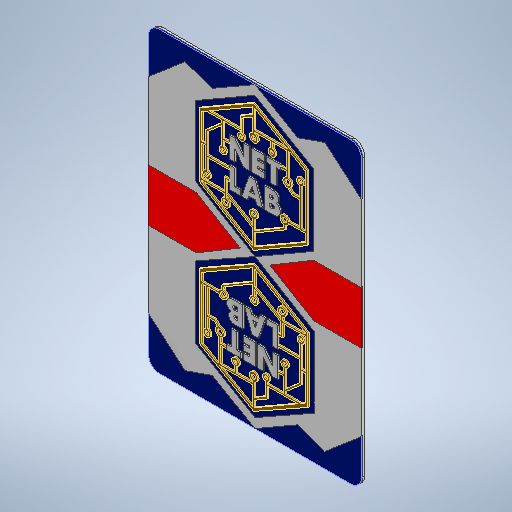
# Autodesk Inventor part: 0ofwifi
Saved by Autodesk Inventor 2025 (Build 290162010, 162A)
## iProperties
Created: 2024-07-12
Part Number: 0ofwifi
Material: Generic
Document SubType Name: Modeling
Designer: joshu
Density: 1 g/cm^3
Appearance: Default
Author: joshu
Autodesk Inventor part; units mm, degrees
(part 1 of 2)
ref_plane "YZ Plane" through (0, 0, 0) normal (1, 0, 0) x (0, 1, 0)
ref_plane "XZ Plane" through (0, 0, 0) normal (0, 1, 0) x (-1, 0, 0)
ref_plane "XY Plane" through (0, 0, 0) normal (0, 0, 1) x (1, 0, 0)
sketch "Sketch1" plane through (0, 0, 0) normal (0, 0, 1) x (1, 0, 0)
  line L0 (0, 0) -> (63.5, 0)
  line L1 (63.5, 0) -> (63.5, 88.9)
  line L2 (63.5, 88.9) -> (0, 88.9)
  line L3 (0, 88.9) -> (0, 0)
  line L4 (31.75, 44.45) -> (49.3079, 54.587)
  line L5 (49.3079, 54.587) -> (49.3079, 75.7826)
  line L6 (49.3079, 75.7826) -> (31.6801, 86.0828)
  line L7 (31.6801, 86.0828) -> (13.967, 75.8563)
  line L8 (13.967, 75.8563) -> (13.967, 55.04)
  line L9 (13.967, 55.04) -> (31.75, 44.45)
  line L10 (15.5263, 74.956) -> (31.6754, 84.2796)
  line L11 (31.6754, 84.2796) -> (47.7487, 74.8877)
  line L12 (47.7487, 74.8877) -> (47.7487, 55.4872)
  line L13 (47.7487, 55.4872) -> (31.7622, 46.2575)
  line L14 (31.7622, 46.2575) -> (15.5263, 55.9263)
  line L15 (15.5263, 55.9263) -> (15.5263, 74.956)
  line L16 (47.1273, 56.0392) -> (31.9379, 47.2671)
  line L17 (31.3664, 47.317) -> (16.2977, 56.192)
  line L18 (41.8086, 77.4972) -> (32.0418, 77.4972)
  line L19 (42.0908, 76.9257) -> (42.0908, 70.0939)
  line L20 (41.5193, 72.1376) -> (39.6994, 72.1376)
  line L21 (39.6994, 72.1376) -> (39.6994, 71.5661)
  line L22 (39.6994, 71.5661) -> (41.5193, 71.5661)
  arc A0 (31.465, 76.5861) -> (32.0365, 76.5861) centre (31.7507, 75.3324) ccw
  arc A1 (36.8763, 75.3571) -> (37.4478, 75.3571) centre (37.162, 74.2504) ccw
  circle A2 centre (37.162, 74.2504) radius 0.4762
  circle A3 centre (31.7507, 75.3324) radius 0.6191
  line L23 (45.9318, 69.8545) -> (45.9318, 58.9507)
  line L24 (45.3603, 66.7769) -> (43.3841, 66.7769)
  line L25 (43.1915, 66.2054) -> (45.3603, 66.2054)
  circle A4 centre (41.805, 68.7917) radius 0.762
  line L26 (43.1915, 66.2054) -> (41.9826, 67.4703)
  line L27 (43.3841, 66.7769) -> (42.5287, 67.6719)
  arc A5 (45.9318, 69.8545) -> (45.3603, 69.8545) centre (45.646, 70.9598) ccw
  circle A6 centre (45.646, 70.9598) radius 0.5715
  line L28 (40.6132, 56.5528) -> (40.6132, 57.4113)
  circle A7 centre (40.899, 58.665) radius 0.7144
  line L29 (32.0418, 83.1688) -> (32.0418, 77.4972)
  line L30 (32.0365, 76.9257) -> (32.0365, 76.5861)
  line L31 (32.0365, 76.9257) -> (36.8763, 76.9257)
  line L32 (36.8763, 75.3571) -> (36.8763, 76.9257)
  line L33 (37.4478, 76.9257) -> (37.4478, 75.3571)
  line L34 (37.4478, 76.9257) -> (41.5193, 76.9257)
  line L35 (42.0908, 76.9257) -> (42.7928, 76.9257)
  line L36 (32.0365, 83.1719) -> (41.8086, 77.4972)
  line L37 (42.7928, 76.9257) -> (47.1273, 74.4086)
  line L38 (41.5193, 70.0939) -> (41.5193, 71.5661)
  line L39 (41.5193, 72.1376) -> (41.5193, 76.9257)
  arc A8 (41.5193, 70.0939) -> (41.9826, 67.4703) centre (41.805, 68.7917) ccw
  arc A9 (42.5287, 67.6719) -> (42.0908, 70.0939) centre (41.805, 68.7917) ccw
  line L40 (45.3603, 58.9507) -> (45.3603, 66.2054)
  line L41 (45.3603, 66.7769) -> (45.3603, 69.8545)
  line L42 (47.1273, 58.9507) -> (45.9318, 58.9507)
  line L43 (45.3603, 58.9507) -> (42.1527, 58.9507)
  line L44 (42.1475, 58.3804) -> (47.1273, 58.3804)
  line L45 (41.1819, 57.4161) -> (41.1819, 56.2658)
  arc A10 (42.1527, 58.9507) -> (40.6132, 57.4113) centre (40.899, 58.665) ccw
  arc A11 (41.1819, 57.4161) -> (42.1475, 58.3804) centre (40.899, 58.665) ccw
  line L46 (47.1273, 74.4086) -> (47.1273, 58.9507)
  line L47 (47.1273, 58.3804) -> (47.1273, 56.0392)
  line L48 (27.6974, 78.6822) -> (27.6974, 79.0777)
  line L49 (28.2689, 78.6822) -> (31.465, 80.528)
  line L50 (27.6974, 79.0777) -> (31.465, 81.2535)
  line L51 (31.465, 76.5861) -> (31.465, 80.528)
  line L52 (31.465, 81.2535) -> (31.465, 83.1596)
  line L53 (31.9379, 51.4601) -> (40.6132, 56.5528)
  line L54 (31.9379, 50.8392) -> (41.1819, 56.2658)
  line L55 (16.2977, 57.1448) -> (22.9994, 57.1448)
  line L56 (22.9994, 56.5733) -> (16.2977, 56.5733)
  line L57 (16.2977, 56.5733) -> (16.2977, 57.1448)
  line L58 (22.9994, 60.9472) -> (23.5709, 60.9472)
  line L59 (22.9994, 60.9472) -> (24.4329, 60.9472)
  line L60 (24.4329, 60.9472) -> (24.4329, 60.3757)
  line L61 (24.4329, 60.3757) -> (23.5709, 60.3757)
  line L62 (22.9994, 60.3757) -> (22.9994, 60.9472)
  line L63 (23.5709, 56.4373) -> (31.3664, 51.9861)
  line L64 (31.3664, 52.5972) -> (23.5709, 57.0484)
  arc A12 (31.9379, 54.3552) -> (31.3664, 54.3552) centre (31.6521, 55.5111) ccw
  circle A13 centre (31.6521, 55.5111) radius 0.6191
  arc A14 (22.9994, 55.5805) -> (23.5709, 55.5805) centre (23.2852, 54.3309) ccw
  circle A15 centre (23.2852, 54.3309) radius 0.7144
  line L65 (23.5709, 60.3757) -> (23.5709, 57.0484)
  line L66 (23.5709, 56.4373) -> (23.5709, 55.5805)
  line L67 (22.9994, 55.5805) -> (22.9994, 56.5733)
  line L68 (22.9994, 57.1448) -> (22.9994, 60.9472)
  line L69 (31.3664, 54.3552) -> (31.3664, 52.5972)
  line L70 (31.3664, 51.9861) -> (31.3664, 47.317)
  line L71 (31.9379, 47.2671) -> (31.9379, 50.8392)
  line L72 (31.9379, 51.4601) -> (31.9379, 54.3552)
  arc A16 (27.6974, 74.6924) -> (28.2689, 74.6924) centre (27.9831, 73.6844) ccw
  circle A17 centre (27.9831, 73.6844) radius 0.4763
  line L73 (18.5492, 75.7007) -> (27.6974, 75.7007)
  line L74 (22.769, 70.6818) -> (24.4329, 70.6818)
  line L75 (24.4329, 70.6818) -> (24.4329, 70.1103)
  line L76 (24.4329, 70.1103) -> (22.769, 70.1103)
  line L77 (22.769, 70.1103) -> (22.769, 70.2009)
  line L78 (16.2977, 66.7769) -> (17.4065, 66.7769)
  line L79 (17.978, 66.7769) -> (17.978, 66.2054)
  line L80 (17.4065, 66.2054) -> (16.2977, 66.2054)
  line L81 (17.978, 63.9706) -> (24.4329, 63.9706)
  line L82 (24.4329, 63.9706) -> (24.4329, 63.3991)
  line L83 (24.4329, 63.3991) -> (17.978, 63.3991)
  line L84 (17.4065, 66.7769) -> (17.4065, 70.2549)
  line L85 (17.978, 70.0307) -> (17.978, 66.7769)
  line L86 (17.4065, 70.2549) -> (22.1975, 74.4365)
  line L87 (17.978, 70.0307) -> (22.1975, 73.7135)
  arc A18 (22.1975, 68.5281) -> (22.769, 68.5281) centre (22.4833, 67.4703) ccw
  circle A19 centre (22.4833, 67.4703) radius 0.5239
  line L88 (16.2977, 74.4004) -> (17.5596, 75.1292)
  line L89 (18.5492, 75.7007) -> (31.465, 83.1596)
  line L90 (27.6974, 75.1292) -> (22.769, 75.1292)
  line L91 (22.1975, 75.1292) -> (17.5596, 75.1292)
  line L92 (22.1975, 74.4365) -> (22.1975, 75.1292)
  line L93 (28.2689, 74.6924) -> (28.2689, 78.6822)
  line L94 (22.769, 75.1292) -> (22.769, 70.6818)
  line L95 (22.769, 70.1103) -> (22.769, 68.5281)
  line L96 (22.1975, 67.8875) -> (22.1975, 67.9094)
  line L97 (22.1975, 68.5281) -> (22.1975, 73.7135)
  line L98 (16.2977, 56.192) -> (16.2977, 66.2054)
  line L99 (16.2977, 66.7769) -> (16.2977, 74.4004)
  line L100 (17.978, 63.9706) -> (17.978, 66.2054)
  line L101 (27.6974, 78.6822) -> (27.6974, 75.7007)
  line L102 (27.6974, 75.1292) -> (27.6974, 74.6924)
  line L103 (24.4329, 66.1976) -> (26.1474, 66.1976)
  line L104 (26.1474, 66.1976) -> (26.1474, 69.7075)
  line L105 (26.1474, 72.4542) -> (24.4329, 72.4542)
  line L106 (24.4329, 72.4542) -> (24.4329, 66.1976)
  line L107 (28.7777, 72.4542) -> (30.4922, 72.4542)
  line L108 (30.4922, 72.4542) -> (30.4922, 66.1976)
  line L109 (30.4922, 66.1976) -> (28.7777, 66.1976)
  line L110 (28.7777, 68.9443) -> (28.7777, 72.4542)
  line L111 (28.7777, 66.1976) -> (26.1474, 69.7075)
  line L112 (26.1474, 72.4542) -> (28.7777, 68.9443)
  line L113 (31.2537, 72.4542) -> (32.9682, 72.4542)
  line L114 (32.9682, 66.1976) -> (31.2537, 66.1976)
  line L115 (31.2537, 66.1976) -> (31.2537, 72.4542)
  line L116 (31.2537, 72.4542) -> (34.8385, 72.4542)
  line L117 (34.8385, 72.4542) -> (34.8385, 70.7397)
  line L118 (34.8385, 70.7397) -> (32.9682, 70.7397)
  line L119 (31.2537, 70.7397) -> (31.2537, 72.4542)
  line L120 (32.9682, 70.0633) -> (34.8385, 70.0633)
  line L121 (34.8385, 70.0633) -> (34.8385, 68.5393)
  line L122 (34.8385, 68.5393) -> (32.9682, 68.5393)
  line L123 (31.2537, 68.5393) -> (31.2537, 70.0633)
  line L124 (31.2537, 66.1976) -> (34.8385, 66.1976)
  line L125 (34.8385, 66.1976) -> (34.8385, 67.9121)
  line L126 (34.8385, 67.9121) -> (32.9682, 67.9121)
  line L127 (31.2537, 67.9121) -> (31.2537, 66.1976)
  line L128 (32.9682, 70.7397) -> (32.9682, 70.0633)
  line L129 (32.9682, 68.5393) -> (32.9682, 67.9121)
  line L130 (39.6994, 72.4422) -> (35.4849, 72.4422)
  line L131 (35.4849, 72.4422) -> (35.4849, 70.9182)
  line L132 (39.6994, 70.9182) -> (39.6994, 72.4422)
  line L133 (38.4466, 70.9182) -> (38.4466, 66.1976)
  line L134 (38.4466, 66.1976) -> (36.7321, 66.1976)
  line L135 (36.7321, 66.1976) -> (36.7321, 70.9182)
  line L136 (36.7321, 70.9182) -> (36.8763, 70.9182)
  line L137 (35.4849, 70.9182) -> (36.7321, 70.9182)
  line L138 (38.4466, 70.9182) -> (39.6994, 70.9182)
  line L139 (24.4329, 64.6461) -> (26.1474, 64.6461)
  line L140 (26.1474, 64.6461) -> (26.1474, 59.9044)
  line L141 (26.1474, 58.3804) -> (24.4329, 58.3804)
  line L142 (24.4329, 58.3804) -> (24.4329, 64.6461)
  line L143 (24.4329, 58.3804) -> (27.8234, 58.3804)
  line L144 (27.8234, 58.3804) -> (27.8234, 59.9044)
  line L145 (27.8234, 59.9044) -> (26.1474, 59.9044)
  line L146 (24.4329, 59.9044) -> (24.4329, 58.3804)
  line L147 (28.1466, 58.3804) -> (29.8611, 58.3804)
  line L148 (29.8611, 58.3804) -> (30.3254, 59.5144)
  line L149 (30.3254, 59.5144) -> (32.2304, 59.5144)
  line L150 (30.3254, 64.6461) -> (32.2304, 64.6461)
  line L151 (28.1466, 58.3804) -> (30.3254, 64.6461)
  line L152 (32.728, 58.3804) -> (34.4425, 58.3804)
  line L153 (32.728, 58.3804) -> (32.2304, 59.5144)
  line L154 (34.4425, 58.3804) -> (32.2304, 64.6461)
  line L155 (30.6203, 60.8236) -> (31.9379, 60.8236)
  line L156 (31.9379, 60.8236) -> (31.2779, 62.4085)
  line L157 (31.2779, 62.4085) -> (30.6203, 60.8236)
  line L158 (34.9216, 58.3804) -> (34.9216, 64.6461)
  line L159 (34.9216, 64.6461) -> (37.8691, 64.6461)
  line L160 (34.9216, 58.3804) -> (37.8691, 58.3804)
  line L161 (36.5599, 59.8143) -> (36.5599, 60.939)
  line L162 (36.5599, 62.1736) -> (36.5599, 63.1944)
  line L163 (36.5599, 63.1944) -> (37.2133, 63.1944)
  line L164 (36.5599, 62.1736) -> (37.2133, 62.1736)
  arc A20 (37.2133, 62.1736) -> (37.2133, 63.1944) centre (37.055, 62.684) ccw
  line L165 (36.5599, 60.939) -> (37.4519, 60.939)
  line L166 (36.5599, 59.8143) -> (37.4396, 59.8143)
  arc A21 (37.4396, 59.8143) -> (37.4519, 60.939) centre (37.3959, 60.3772) ccw
  arc A22 (38.5631, 61.7817) -> (37.8691, 64.6461) centre (37.5266, 63.0469) ccw
  arc A23 (37.8691, 58.3804) -> (38.5631, 61.7817) centre (37.9604, 60.1332) ccw
  arc A24 (17.4065, 59.8724) -> (17.978, 59.8724) centre (17.6923, 58.815) ccw
  circle A25 centre (17.6923, 58.815) radius 0.5239
  line L167 (17.4065, 66.2054) -> (17.4065, 59.8724)
  line L168 (17.978, 59.8724) -> (17.978, 63.3991)
  line L169 (32.0418, 83.1688) -> (41.8086, 77.4972)
  line L170 (32.0418, 77.4972) -> (41.8086, 77.4972)
  line L171 (32.0418, 77.4972) -> (32.0418, 83.1688)
  line L172 (0, 44.45) -> (63.5, 44.45) construction
  line L173 (31.75, 88.9) -> (31.75, 0) construction
  line L174 (0, 52.2573) -> (14.2102, 52.2573)
  line L175 (14.2102, 52.2573) -> (27.3204, 44.45)
  line L176 (0, 36.6427) -> (14.2102, 36.6427)
  line L177 (14.2102, 36.6427) -> (27.3204, 44.45)
  line L178 (63.5, 52.2573) -> (49.2898, 52.2573)
  line L179 (49.2898, 52.2573) -> (36.1796, 44.45)
  line L180 (49.2898, 36.6427) -> (36.1796, 44.45)
  line L181 (63.5, 36.6427) -> (49.2898, 36.6427)
  line L182 (0, 75.0796) -> (10.8905, 84.3747)
  line L183 (10.8905, 84.3747) -> (18.9583, 81.5148)
  line L184 (18.9583, 81.5148) -> (31.75, 88.9)
  line L185 (63.5, 75.0796) -> (52.6095, 84.3747)
  line L186 (52.6095, 84.3747) -> (44.5417, 81.5148)
  line L187 (44.5417, 81.5148) -> (31.75, 88.9)
  line L188 (46.0393, 22.6946) -> (47.1481, 22.6946)
  line L189 (45.4678, 22.1231) -> (45.4678, 22.6946)
  line L190 (45.4678, 24.9294) -> (45.4678, 22.6946)
  line L191 (47.1481, 22.1231) -> (46.0393, 22.1231)
  line L192 (47.1481, 32.3267) -> (47.1481, 31.7552)
  line L193 (47.1481, 32.708) -> (47.1481, 22.6946)
  line L194 (47.1481, 31.7552) -> (40.4464, 31.7552)
  line L195 (40.4464, 32.3267) -> (47.1481, 32.3267)
  line L196 (45.4678, 29.0276) -> (45.4678, 25.5009)
  line L197 (46.0393, 22.6946) -> (46.0393, 29.0276)
  circle A26 centre (45.7535, 30.085) radius 0.5239
  arc A27 (46.0393, 29.0276) -> (45.4678, 29.0276) centre (45.7535, 30.085) ccw
  line L198 (20.6531, 11.9743) -> (16.3185, 14.4914)
  line L199 (21.355, 11.9743) -> (20.6531, 11.9743)
  line L200 (21.9265, 16.7624) -> (21.9265, 11.9743)
  line L201 (21.355, 11.9743) -> (21.355, 18.8061)
  line L202 (21.9265, 16.7624) -> (23.7464, 16.7624)
  line L203 (23.7464, 17.3339) -> (21.9265, 17.3339)
  line L204 (25.998, 11.9743) -> (21.9265, 11.9743)
  line L205 (26.5695, 13.5429) -> (26.5695, 11.9743)
  circle A28 centre (21.6408, 20.1083) radius 0.762
  circle A29 centre (26.2838, 14.6496) radius 0.4762
  arc A30 (26.5695, 13.5429) -> (25.998, 13.5429) centre (26.2838, 14.6496) ccw
  line L206 (31.4093, 11.9743) -> (26.5695, 11.9743)
  arc A31 (31.9808, 12.3139) -> (31.4093, 12.3139) centre (31.6951, 13.5676) ccw
  line L207 (25.998, 11.9743) -> (25.998, 13.5429)
  line L208 (45.4678, 24.9294) -> (39.013, 24.9294)
  line L209 (39.013, 25.5009) -> (45.4678, 25.5009)
  line L210 (39.013, 24.9294) -> (39.013, 25.5009)
  circle A32 centre (40.1606, 34.5691) radius 0.7144
  arc A33 (40.4464, 33.3195) -> (39.8749, 33.3195) centre (40.1606, 34.5691) ccw
  line L211 (39.8749, 32.4627) -> (39.8749, 33.3195)
  line L212 (40.4464, 33.3195) -> (40.4464, 32.3267)
  line L213 (39.013, 27.9528) -> (39.013, 28.5243)
  line L214 (39.8749, 28.5243) -> (39.8749, 31.8516)
  line L215 (39.013, 28.5243) -> (39.8749, 28.5243)
  line L216 (40.4464, 31.7552) -> (40.4464, 27.9528)
  line L217 (40.4464, 28.5243) -> (40.4464, 27.9528)
  line L218 (40.4464, 27.9528) -> (39.8749, 27.9528)
  line L219 (40.4464, 27.9528) -> (39.013, 27.9528)
  line L220 (33.5847, 30.5196) -> (33.1204, 29.3856)
  line L221 (35.6224, 28.9956) -> (37.2985, 28.9956)
  line L222 (35.2992, 30.5196) -> (33.5847, 30.5196)
  line L223 (39.013, 28.9956) -> (39.013, 30.5196)
  line L224 (35.2992, 30.5196) -> (33.1204, 24.2539)
  line L225 (46.0393, 18.6451) -> (41.2483, 14.4635)
  line L226 (45.4678, 18.8693) -> (41.2483, 15.1865)
  line L227 (40.6768, 18.7897) -> (40.6768, 20.3719)
  line L228 (41.2483, 21.0125) -> (41.2483, 20.9906)
  line L229 (41.2483, 20.3719) -> (41.2483, 15.1865)
  line L230 (40.6768, 13.7708) -> (40.6768, 18.2182)
  line L231 (41.2483, 14.4635) -> (41.2483, 13.7708)
  line L232 (41.2483, 13.7708) -> (45.8862, 13.7708)
  line L233 (47.1481, 22.1231) -> (47.1481, 14.4996)
  line L234 (47.1481, 14.4996) -> (45.8862, 13.7708)
  circle A34 centre (40.9626, 21.4297) radius 0.5239
  line L235 (32.8255, 28.0764) -> (31.5079, 28.0764)
  line L236 (32.1679, 26.4915) -> (32.8255, 28.0764)
  line L237 (31.5079, 28.0764) -> (32.1679, 26.4915)
  line L238 (33.1204, 29.3856) -> (31.2154, 29.3856)
  line L239 (35.6224, 30.5196) -> (35.6224, 28.9956)
  line L240 (37.2985, 24.2539) -> (37.2985, 28.9956)
  line L241 (37.2985, 30.5196) -> (39.013, 30.5196)
  line L242 (39.013, 30.5196) -> (39.013, 24.2539)
  line L243 (39.013, 30.5196) -> (35.6224, 30.5196)
  line L244 (39.013, 24.2539) -> (37.2985, 24.2539)
  line L245 (33.1204, 24.2539) -> (31.2154, 24.2539)
  line L246 (30.7178, 30.5196) -> (31.2154, 29.3856)
  line L247 (37.2985, 16.4458) -> (39.013, 16.4458)
  line L248 (40.6768, 18.2182) -> (39.013, 18.2182)
  line L249 (39.013, 18.7897) -> (40.6768, 18.7897)
  line L250 (40.6768, 18.7897) -> (40.6768, 18.6991)
  line L251 (39.013, 18.2182) -> (39.013, 18.7897)
  line L252 (46.0393, 22.1231) -> (46.0393, 18.6451)
  line L253 (45.4678, 18.8693) -> (45.4678, 22.1231)
  arc A35 (41.2483, 20.3719) -> (40.6768, 20.3719) centre (40.9626, 21.4297) ccw
  line L254 (39.013, 16.4458) -> (39.013, 22.7024)
  line L255 (39.013, 22.7024) -> (37.2985, 22.7024)
  line L256 (32.9536, 22.7024) -> (34.6681, 22.7024)
  line L257 (30.4777, 22.7024) -> (32.1922, 22.7024)
  line L258 (30.4777, 18.8367) -> (28.6073, 18.8367)
  line L259 (32.1922, 22.7024) -> (28.6073, 22.7024)
  line L260 (28.6073, 22.7024) -> (28.6073, 20.9879)
  line L261 (28.6073, 20.9879) -> (30.4777, 20.9879)
  line L262 (32.1922, 20.9879) -> (32.1922, 22.7024)
  line L263 (30.4777, 20.3607) -> (30.4777, 20.9879)
  line L264 (28.6073, 20.3607) -> (30.4777, 20.3607)
  line L265 (28.6073, 18.8367) -> (28.6073, 20.3607)
  line L266 (32.1922, 20.3607) -> (32.1922, 18.8367)
  line L267 (30.4777, 18.1603) -> (30.4777, 18.8367)
  line L268 (26.8859, 25.7056) -> (26.2325, 25.7056)
  line L269 (26.8859, 29.0857) -> (26.0062, 29.0857)
  line L270 (26.8859, 27.961) -> (25.9939, 27.961)
  line L271 (28.5242, 30.5196) -> (25.5767, 30.5196)
  line L272 (32.0794, 36.9139) -> (32.0794, 41.583)
  line L273 (31.5079, 41.6329) -> (31.5079, 38.0608)
  line L274 (26.8859, 26.7264) -> (26.8859, 25.7056)
  line L275 (28.5242, 24.2539) -> (25.5767, 24.2539)
  line L276 (29.0033, 30.5196) -> (31.2154, 24.2539)
  line L277 (30.7178, 30.5196) -> (29.0033, 30.5196)
  line L278 (26.8859, 26.7264) -> (26.2325, 26.7264)
  line L279 (28.5242, 30.5196) -> (28.5242, 24.2539)
  arc A36 (26.2325, 26.7264) -> (26.2325, 25.7056) centre (26.3908, 26.216) ccw
  line L280 (26.8859, 29.0857) -> (26.8859, 27.961)
  arc A37 (26.0062, 29.0857) -> (25.9939, 27.961) centre (26.0499, 28.5228) ccw
  arc A38 (24.8827, 27.1183) -> (25.5767, 24.2539) centre (25.9192, 25.8531) ccw
  arc A39 (25.5767, 30.5196) -> (24.8827, 27.1183) centre (25.4854, 28.7668) ccw
  line L281 (23.7464, 16.7624) -> (23.7464, 17.3339)
  line L282 (24.9992, 22.7024) -> (26.7137, 22.7024)
  line L283 (27.961, 17.9818) -> (26.7137, 17.9818)
  line L284 (26.7137, 22.7024) -> (26.7137, 17.9818)
  line L285 (26.7137, 17.9818) -> (26.5695, 17.9818)
  line L286 (24.9992, 17.9818) -> (24.9992, 22.7024)
  line L287 (24.9992, 17.9818) -> (23.7464, 17.9818)
  line L288 (27.961, 16.4578) -> (27.961, 17.9818)
  line L289 (23.7464, 16.4578) -> (27.961, 16.4578)
  line L290 (23.7464, 17.9818) -> (23.7464, 16.4578)
  line L291 (31.75, 44.45) -> (14.1379, 34.5158)
  line L292 (15.6972, 33.6051) -> (31.7276, 42.6471)
  line L293 (16.3185, 32.8608) -> (31.5079, 41.6329)
  line L294 (31.5079, 37.4399) -> (22.8326, 32.3472)
  line L295 (31.5079, 38.0608) -> (22.2639, 32.6342)
  line L296 (31.5079, 37.4399) -> (31.5079, 34.5448)
  line L297 (35.7484, 10.2178) -> (35.7484, 9.8223)
  line L298 (35.1769, 10.2178) -> (31.9808, 8.372)
  line L299 (35.7484, 9.8223) -> (31.9808, 7.6465)
  line L300 (31.9808, 12.3139) -> (31.9808, 8.372)
  line L301 (31.9808, 7.6465) -> (31.9808, 5.7404)
  circle A40 centre (35.4627, 15.2156) radius 0.4763
  arc A41 (35.7484, 14.2076) -> (35.1769, 14.2076) centre (35.4627, 15.2156) ccw
  line L302 (35.7484, 13.7708) -> (35.7484, 14.2076)
  line L303 (35.7484, 13.7708) -> (40.6768, 13.7708)
  line L304 (44.8966, 13.1993) -> (35.7484, 13.1993)
  line L305 (35.1769, 14.2076) -> (35.1769, 10.2178)
  line L306 (35.7484, 10.2178) -> (35.7484, 13.1993)
  line L307 (44.8966, 13.1993) -> (31.9808, 5.7404)
  line L308 (31.4093, 11.9743) -> (31.4093, 12.3139)
  line L309 (47.9195, 13.7706) -> (31.7623, 4.657)
  circle A42 centre (31.6951, 13.5676) radius 0.6191
  line L310 (31.7499, 2.8598) -> (49.4788, 12.8599)
  line L311 (47.9195, 32.9751) -> (47.9195, 13.7706)
  line L312 (49.4788, 12.8599) -> (49.4788, 33.86)
  circle A43 centre (31.7937, 33.3889) radius 0.6191
  line L313 (32.0794, 41.583) -> (47.1481, 32.708)
  line L314 (49.4788, 33.86) -> (31.75, 44.45)
  line L315 (31.7276, 42.6471) -> (47.9195, 32.9751)
  line L316 (32.0794, 36.3028) -> (39.8749, 31.8516)
  line L317 (39.8749, 32.4627) -> (32.0794, 36.9139)
  line L318 (32.0794, 34.5448) -> (32.0794, 36.3028)
  arc A44 (31.5079, 34.5448) -> (32.0794, 34.5448) centre (31.7937, 33.3889) ccw
  circle A45 centre (17.7998, 17.9402) radius 0.5715
  line L319 (18.0855, 22.1231) -> (20.0617, 22.1231)
  line L320 (20.2543, 22.6946) -> (18.0855, 22.6946)
  line L321 (22.8326, 32.3472) -> (22.8326, 31.4887)
  circle A46 centre (22.5468, 30.235) radius 0.7144
  line L322 (21.2984, 30.5196) -> (16.3185, 30.5196)
  line L323 (22.2639, 31.4839) -> (22.2639, 32.6342)
  arc A47 (21.2931, 29.9493) -> (22.8326, 31.4887) centre (22.5468, 30.235) ccw
  arc A48 (22.2639, 31.4839) -> (21.2984, 30.5196) centre (22.5468, 30.235) ccw
  line L324 (16.3185, 30.5196) -> (16.3185, 32.8608)
  line L325 (14.1379, 34.5158) -> (14.1379, 13.1174)
  line L326 (15.6972, 14.0137) -> (15.6972, 33.6051)
  line L327 (17.514, 19.0455) -> (17.514, 29.9493)
  line L328 (20.2543, 22.6946) -> (21.4633, 21.4297)
  line L329 (20.0617, 22.1231) -> (20.9171, 21.2281)
  arc A49 (17.514, 19.0455) -> (18.0855, 19.0455) centre (17.7998, 17.9402) ccw
  line L330 (21.9265, 18.8061) -> (21.9265, 17.3339)
  arc A50 (20.9171, 21.2281) -> (21.355, 18.8061) centre (21.6408, 20.1083) ccw
  line L331 (18.0855, 22.1231) -> (18.0855, 19.0455)
  line L332 (16.3185, 14.4914) -> (16.3185, 29.9493)
  line L333 (16.3185, 29.9493) -> (17.514, 29.9493)
  line L334 (18.0855, 29.9493) -> (18.0855, 22.6946)
  line L335 (18.0855, 29.9493) -> (21.2931, 29.9493)
  arc A51 (21.9265, 18.8061) -> (21.4633, 21.4297) centre (21.6408, 20.1083) ccw
  line L336 (14.1379, 13.1174) -> (31.7499, 2.8598)
  line L337 (31.7623, 4.657) -> (15.6972, 14.0137)
  line L338 (21.6372, 11.4028) -> (31.404, 11.4028)
  line L339 (31.404, 11.4028) -> (31.404, 5.7312)
  line L340 (31.404, 5.7312) -> (21.6372, 11.4028)
  line L341 (37.2985, 22.7024) -> (37.2985, 19.1925)
  line L342 (34.6681, 16.4458) -> (32.9536, 16.4458)
  line L343 (32.9536, 16.4458) -> (32.9536, 22.7024)
  line L344 (34.6681, 22.7024) -> (37.2985, 19.1925)
  line L345 (28.6073, 18.1603) -> (30.4777, 18.1603)
  line L346 (32.1922, 16.4458) -> (28.6073, 16.4458)
  line L347 (28.6073, 16.4458) -> (28.6073, 18.1603)
  line L348 (32.1922, 22.7024) -> (32.1922, 16.4458)
  line L349 (32.1922, 16.4458) -> (30.4777, 16.4458)
  line L350 (34.6681, 19.9557) -> (34.6681, 16.4458)
  line L351 (37.2985, 16.4458) -> (34.6681, 19.9557)
  line L352 (32.1922, 18.1603) -> (32.1922, 16.4458)
  line L353 (0, 13.8204) -> (10.8905, 4.5253)
  line L354 (10.8905, 4.5253) -> (18.9583, 7.3852)
  line L355 (18.9583, 7.3852) -> (31.75, 0)
  line L356 (63.5, 13.8204) -> (52.6095, 4.5253)
  line L357 (52.6095, 4.5253) -> (44.5417, 7.3852)
  line L358 (44.5417, 7.3852) -> (31.75, 0)
  point P0 (31.9379, 47.317)
  point P1 (31.7229, 65.2666)
  point P2 (31.7229, 23.6334)
  point P3 (31.7229, 23.6334)
  point P4 (31.9379, 5.6837)
  point P5 (63.5, 75.0796)
  dimension "d0" = 63.5
  dimension "d1" = 88.9
  dimension "d43" = 44.45
  dimension "d99" = 120
  constraints: 718 end point, 170 parallel, 64 point on circle, 50 centre point, 42 perpendicular, 36 horizontal, 21 point on line, 20 coincident, 19 symmetric about line, 7 collinear, 5 midpoint, 4 vertical, 17 other
  measures "d0" distance of L2.end L1.end
  measures "d1" distance of L1.end L0.end
  measures "d43" distance between parallel lines of L172 L2
  measures "d99" angle of L357 L356
extrude "Extrusion1" add sketch "Sketch1" along normal blind 0.4 contours L3 L353 L354 L355 L0 | L358 L357 L356 L1 L0 | L3 L2 L184 L183 L182 | L185 L186 L187 L2 L1 | L9 L8 L7 L6 L5 L4 | L314 L312 L310 L336 L325 L291 | L10 L11 L12 L13 L14 L15 | L16 L71 L54 L45 A11 L44 L47 | L17 L98 L56 L67 A14 L66 L63 L70 | L18 L29 L36 | L35 L37 L46 L42 L23 A5 L41 L24 L27 A9 L19 | L20 L132 L130 L131 L137 L135 L134 L133 L138 L22 L38 A8 L26 L25 L40 L43 A10 L28 L53 L72 A12 L69 L64 L65 L61 L142 L141 L143 L144 L145 L140 L139 L81 L100 L79 L85 L87 L97 A18 L95 L76 L106 L103 L104 L111 L109 L108 L107 L110 L112 L105 L74 L94 L90 L102 A16 L93 L49 L51 A0 L30 L31 L32 A1 L33 L34 L39 | L21 L132 L138 L133 L134 L135 L137 L131 L130 | L106 L105 L112 L110 L107 L108 L109 L111 L104 L103 L75 | L60 L142 L82 L139 L140 L145 L144 L143 L141 | L59 L58 L62 L68 L55 L98 L80 L167 A24 L168 L83 L142 | A2 | A3 | A4 | A6 | A7 | L101 L73 L89 L52 L50 L48 | A13 | A15 | A17 | L99 L88 L91 L92 L86 L84 L78 | A19 | L113 L116 L117 L118 L128 L120 L121 L122 L129 L126 L125 L124 L114 L115 | L151 L150 L154 L152 L153 L149 L148 L147 | L157 L156 L155 | L158 L159 A22 A23 L160 | L161 L165 A21 L166 | L162 L163 A20 L164 | A25 | L197 A27 L196 L209 L242 L219 L218 L216 L194 L193 L188 | L210 L242 L244 L240 L221 L239 L243 L241 L223 L213 | L208 L190 L189 L253 L226 L229 A35 L227 L249 L254 L255 L341 L344 L256 L343 L342 L350 L351 L247 L248 L230 L303 L302 A41 L305 L298 L300 A31 L308 L206 L205 A30 L207 L204 L200 L202 L290 L289 L288 L283 L284 L282 L286 L287 L203 L330 A51 L328 L320 L334 L335 A47 L321 L294 L296 A44 L318 L316 L214 L215 L242 L223 L241 L243 L239 L221 L240 L244 | L251 L254 L247 L351 L350 L342 L343 L256 L344 L341 L255 | L290 L287 L286 L282 L284 L283 L288 L289 L281 | L233 L234 L232 L231 L225 L252 L191 | L193 L195 L212 A33 L211 L317 L272 L313 | A26 | L198 L332 L333 L327 A49 L331 L319 L329 A50 L201 L199 | A28 | A29 | A32 | L222 L224 L245 L276 L277 L246 L238 L220 | A34 | L236 L237 L235 | L257 L262 L348 L266 L346 L347 L345 L267 L258 L265 L264 L263 L261 L260 L259 | L268 A36 L278 L274 | L280 L270 A37 L269 | L279 L275 A38 A39 L271 | L273 L295 L323 A48 L322 L324 L293 | L292 L315 L311 L309 L337 L326 | L306 L304 L307 L301 L299 L297 | A40 | A42 | A43 | A45 | A46 | L338 L339 L340
extrude "Extrusion12" add sketch "Sketch1" along normal blind 0.4 separate body contours L3 L174 L175 L177 L176 | L181 L180 L179 L178 L1
extrude "Extrusion13" add sketch "Sketch1" along normal blind 0.4 separate body contours L355 L354 L353 L3 L176 L177 L175 L174 L182 L183 L184 L187 L186 L185 L1 L178 L179 L180 L181 L356 L357 L358
extrude "Extrusion14" add sketch "Sketch1" against normal blind 0.4 contours L21 L132 L138 L133 L134 L135 L137 L131 L130 | L106 L105 L112 L110 L107 L108 L109 L111 L104 L103 L75 | L60 L142 L82 L139 L140 L145 L144 L143 L141 | L113 L116 L117 L118 L128 L120 L121 L122 L129 L126 L125 L124 L114 L115 | L151 L150 L154 L152 L153 L149 L148 L147 | L158 L159 A22 A23 L160 | L210 L242 L244 L240 L221 L239 L243 L241 L223 L213 | L251 L254 L247 L351 L350 L342 L343 L256 L344 L341 L255 | L290 L287 L286 L282 L284 L283 L288 L289 L281 | L222 L224 L245 L276 L277 L246 L238 L220 | L257 L262 L348 L266 L346 L347 L345 L267 L258 L265 L264 L263 L261 L260 L259 | L279 L275 A38 A39 L271 bodies 3
extrude "Extrusion15" add sketch "Sketch1" against normal blind 0.4 separate body contours L10 L11 L12 L13 L14 L15 | L292 L315 L311 L309 L337 L326
pattern_linear "Rectangular Pattern1" count 2 spacing 0.8 along (0, 0, 1) of "Extrusion15" bodies 4
pattern_linear "Rectangular Pattern2" count 2 spacing 0.8 along (0, 0, 1) of "Extrusion14" bodies 3
extrude "Extrusion16" cut sketch "Sketch1" against normal blind 0.4 contours L9 L8 L7 L6 L5 L4 | L314 L312 L310 L336 L325 L291 | L10 L11 L12 L13 L14 L15 | L16 L71 L54 L45 A11 L44 L47 | L17 L98 L56 L67 A14 L66 L63 L70 | L18 L29 L36 | L35 L37 L46 L42 L23 A5 L41 L24 L27 A9 L19 | L20 L132 L130 L131 L137 L135 L134 L133 L138 L22 L38 A8 L26 L25 L40 L43 A10 L28 L53 L72 A12 L69 L64 L65 L61 L142 L141 L143 L144 L145 L140 L139 L81 L100 L79 L85 L87 L97 A18 L95 L76 L106 L103 L104 L111 L109 L108 L107 L110 L112 L105 L74 L94 L90 L102 A16 L93 L49 L51 A0 L30 L31 L32 A1 L33 L34 L39 | L21 L132 L138 L133 L134 L135 L137 L131 L130 | L106 L105 L112 L110 L107 L108 L109 L111 L104 L103 L75 | L60 L142 L82 L139 L140 L145 L144 L143 L141 | L59 L58 L62 L68 L55 L98 L80 L167 A24 L168 L83 L142 | A2 | A3 | A4 | A6 | A7 | L101 L73 L89 L52 L50 L48 | A13 | A15 | A17 | L99 L88 L91 L92 L86 L84 L78 | A19 | L113 L116 L117 L118 L128 L120 L121 L122 L129 L126 L125 L124 L114 L115 | L151 L150 L154 L152 L153 L149 L148 L147 | L157 L156 L155 | L158 L159 A22 A23 L160 | L161 L165 A21 L166 | L162 L163 A20 L164 | A25 | L197 A27 L196 L209 L242 L219 L218 L216 L194 L193 L188 | L210 L242 L244 L240 L221 L239 L243 L241 L223 L213 | L208 L190 L189 L253 L226 L229 A35 L227 L249 L254 L255 L341 L344 L256 L343 L342 L350 L351 L247 L248 L230 L303 L302 A41 L305 L298 L300 A31 L308 L206 L205 A30 L207 L204 L200 L202 L290 L289 L288 L283 L284 L282 L286 L287 L203 L330 A51 L328 L320 L334 L335 A47 L321 L294 L296 A44 L318 L316 L214 L215 L242 L223 L241 L243 L239 L221 L240 L244 | L251 L254 L247 L351 L350 L342 L343 L256 L344 L341 L255 | L290 L287 L286 L282 L284 L283 L288 L289 L281 | L233 L234 L232 L231 L225 L252 L191 | L193 L195 L212 A33 L211 L317 L272 L313 | A26 | L198 L332 L333 L327 A49 L331 L319 L329 A50 L201 L199 | A28 | A29 | A32 | L222 L224 L245 L276 L277 L246 L238 L220 | A34 | L236 L237 L235 | L257 L262 L348 L266 L346 L347 L345 L267 L258 L265 L264 L263 L261 L260 L259 | L268 A36 L278 L274 | L280 L270 A37 L269 | L279 L275 A38 A39 L271 | L273 L295 L323 A48 L322 L324 L293 | L292 L315 L311 L309 L337 L326 | L306 L304 L307 L301 L299 L297 | A40 | A42 | A43 | A45 | A46 | L338 L339 L340 bodies 3
extrude "Extrusion17" cut sketch "Sketch1" against normal blind 25.4 contours L9 L8 L7 L6 L5 L4 | L314 L312 L310 L336 L325 L291 | L10 L11 L12 L13 L14 L15 | L16 L71 L54 L45 A11 L44 L47 | L17 L98 L56 L67 A14 L66 L63 L70 | L18 L29 L36 | L35 L37 L46 L42 L23 A5 L41 L24 L27 A9 L19 | L20 L132 L130 L131 L137 L135 L134 L133 L138 L22 L38 A8 L26 L25 L40 L43 A10 L28 L53 L72 A12 L69 L64 L65 L61 L142 L141 L143 L144 L145 L140 L139 L81 L100 L79 L85 L87 L97 A18 L95 L76 L106 L103 L104 L111 L109 L108 L107 L110 L112 L105 L74 L94 L90 L102 A16 L93 L49 L51 A0 L30 L31 L32 A1 L33 L34 L39 | L21 L132 L138 L133 L134 L135 L137 L131 L130 | L106 L105 L112 L110 L107 L108 L109 L111 L104 L103 L75 | L60 L142 L82 L139 L140 L145 L144 L143 L141 | L59 L58 L62 L68 L55 L98 L80 L167 A24 L168 L83 L142 | A2 | A3 | A4 | A6 | A7 | L101 L73 L89 L52 L50 L48 | A13 | A15 | A17 | L99 L88 L91 L92 L86 L84 L78 | A19 | L113 L116 L117 L118 L128 L120 L121 L122 L129 L126 L125 L124 L114 L115 | L151 L150 L154 L152 L153 L149 L148 L147 | L157 L156 L155 | L158 L159 A22 A23 L160 | L161 L165 A21 L166 | L162 L163 A20 L164 | A25 | L197 A27 L196 L209 L242 L219 L218 L216 L194 L193 L188 | L210 L242 L244 L240 L221 L239 L243 L241 L223 L213 | L208 L190 L189 L253 L226 L229 A35 L227 L249 L254 L255 L341 L344 L256 L343 L342 L350 L351 L247 L248 L230 L303 L302 A41 L305 L298 L300 A31 L308 L206 L205 A30 L207 L204 L200 L202 L290 L289 L288 L283 L284 L282 L286 L287 L203 L330 A51 L328 L320 L334 L335 A47 L321 L294 L296 A44 L318 L316 L214 L215 L242 L223 L241 L243 L239 L221 L240 L244 | L251 L254 L247 L351 L350 L342 L343 L256 L344 L341 L255 | L290 L287 L286 L282 L284 L283 L288 L289 L281 | L233 L234 L232 L231 L225 L252 L191 | L193 L195 L212 A33 L211 L317 L272 L313 | A26 | L198 L332 L333 L327 A49 L331 L319 L329 A50 L201 L199 | A28 | A29 | A32 | L222 L224 L245 L276 L277 L246 L238 L220 | A34 | L236 L237 L235 | L257 L262 L348 L266 L346 L347 L345 L267 L258 L265 L264 L263 L261 L260 L259 | L268 A36 L278 L274 | L280 L270 A37 L269 | L279 L275 A38 A39 L271 | L273 L295 L323 A48 L322 L324 L293 | L292 L315 L311 L309 L337 L326 | L306 L304 L307 L301 L299 L297 | A40 | A42 | A43 | A45 | A46 | L338 L339 L340 bodies 4
sketch "Sketch14" plane through (0, 0, 0) normal (0, 0, -1) x (-1, 0, 0)
  line L0 (-63.5, 75.0796) -> (-63.5, 88.9) projected
  line L1 (0, 0) -> (-63.5, 0)
  line L2 (-63.5, 0) -> (-63.5, 88.9)
  line L3 (-63.5, 88.9) -> (0, 88.9)
  line L4 (0, 88.9) -> (0, 0)
  line L5 (-62.5, 1) -> (-1, 1)
  line L6 (-1, 1) -> (-1, 87.9)
  line L7 (-1, 87.9) -> (-62.5, 87.9)
  line L8 (-62.5, 87.9) -> (-62.5, 1)
  dimension "d90" = 1
  constraints: 16 end point, 4 parallel, 2 perpendicular, 1 horizontal, 3 other
  measures "d90" distance between parallel lines of L1 L5
extrude "Extrusion18" add sketch "Sketch14" along normal blind 0.2 separate body contours L8 L7 L6 L5
sketch "Sketch16" plane through (0, 0, 0) normal (0, 0, -1) x (-1, 0, 0)
  line L0 (-1, 1) -> (-1, 87.9) projected
  line L1 (-1, 87.9) -> (-62.5, 87.9) projected
  line L2 (-62.5, 87.9) -> (-62.5, 1) projected
  line L3 (-62.5, 1) -> (-1, 1) projected
  line L4 (0, 88.9) -> (0, 75.0796) projected
  line L5 (-31.75, 0) -> (-63.5, 0) projected
  line L6 (0, 88.9) -> (-63.5, 88.9)
  line L7 (-63.5, 88.9) -> (-63.5, 0)
  line L8 (-63.5, 0) -> (0, 0)
  line L9 (0, 0) -> (0, 88.9)
  constraints: 8 end point, 2 parallel, 1 horizontal, 1 perpendicular
extrude "Extrusion19" add sketch "Sketch16" along normal blind 0.2 bodies 3
sketch "Sketch17" plane through (0, 0, -0.2) normal (0, 0, -1) x (-1, 0, 0)
  line L0 (-63.5, 88.9) -> (-63.5, 0)
  line L1 (-63.5, 0) -> (0, 0)
  line L2 (0, 0) -> (0, 88.9)
  line L3 (0, 88.9) -> (-63.5, 88.9)
  line L4 (-62.5, 1) -> (-62.5, 87.9) construction
  line L5 (-62.5, 44.45) -> (-1, 44.45) construction
  line L6 (-1, 87.9) -> (-1, 1) construction
  line L7 (-57.9556, 87.392) -> (-49.5403, 87.392) construction
  line L8 (-49.5403, 87.392) -> (-49.5403, 73.7102) construction
  line L9 (-49.5403, 73.7102) -> (-57.9556, 73.7102) construction
  line L10 (-57.9556, 73.7102) -> (-57.9556, 87.392) construction
  line L11 (-5.5444, 1.508) -> (-13.9597, 1.508) construction
  line L12 (-13.9597, 1.508) -> (-13.9597, 15.8789) construction
  line L13 (-13.9597, 15.8789) -> (-5.5444, 15.8789) construction
  line L14 (-5.5444, 15.8789) -> (-5.5444, 1.508) construction
  line L15 (-62.5, 87.9) -> (-1, 87.9) projected
  line L16 (-1, 1) -> (-62.5, 1) projected
  arc A0 (-54.2587, 71.8195) -> (-55.2164, 71.6633) centre (-53.721, 65.5053) ccw
  arc A1 (-55.2164, 71.6633) -> (-56.1281, 71.3638) centre (-53.7854, 65.7705) ccw
  arc A2 (-56.1281, 71.3638) -> (-56.9803, 70.9245) centre (-53.7898, 65.7811) ccw
  arc A3 (-56.9803, 70.9245) -> (-57.761, 70.3525) centre (-53.6689, 65.5862) ccw
  arc A4 (-57.761, 70.3525) -> (-57.9303, 70.1998) centre (-54.7143, 66.8038) ccw
  arc A5 (-57.9303, 70.1998) -> (-58.1244, 70.0106) centre (-51.5447, 63.4568) ccw
  arc A6 (-58.1244, 70.0106) -> (-58.3037, 69.8254) centre (-51.7023, 63.6139) ccw
  arc A7 (-58.3037, 69.8254) -> (-58.4189, 69.6921) centre (-56.7958, 68.4066) ccw
  line L17 (-58.4189, 69.6921) -> (-58.4764, 69.6194)
  line L18 (-58.4764, 69.6194) -> (-58.0951, 69.2684)
  line L19 (-58.0951, 69.2684) -> (-57.7138, 68.9174)
  line L20 (-57.7138, 68.9174) -> (-57.6118, 69.0338)
  arc A8 (-57.0139, 69.616) -> (-57.6118, 69.0338) centre (-53.6679, 65.5813) ccw
  arc A9 (-56.3308, 70.0963) -> (-57.0139, 69.616) centre (-53.6618, 65.5739) ccw
  arc A10 (-55.5869, 70.4582) -> (-56.3308, 70.0963) centre (-53.7111, 65.6576) ccw
  arc A11 (-54.8079, 70.6887) -> (-55.5869, 70.4582) centre (-53.8421, 65.9928) ccw
  arc A12 (-54.2943, 70.7669) -> (-54.8079, 70.6887) centre (-53.7974, 65.7752) ccw
  arc A13 (-53.7678, 70.793) -> (-54.2943, 70.7669) centre (-53.7678, 65.4777) ccw
  arc A14 (-53.2413, 70.7669) -> (-53.7678, 70.793) centre (-53.7678, 65.4777) ccw
  arc A15 (-52.7277, 70.6887) -> (-53.2413, 70.7669) centre (-53.7382, 65.7752) ccw
  arc A16 (-51.9486, 70.4585) -> (-52.7277, 70.6887) centre (-53.6976, 65.9726) ccw
  arc A17 (-51.2067, 70.0979) -> (-51.9486, 70.4585) centre (-53.8074, 65.6909) ccw
  arc A18 (-50.5247, 69.6182) -> (-51.2067, 70.0979) centre (-53.8645, 65.5942) ccw
  arc A19 (-49.9239, 69.034) -> (-50.5247, 69.6182) centre (-53.9323, 65.5125) ccw
  line L21 (-49.9239, 69.034) -> (-49.8218, 68.9178)
  line L22 (-49.8218, 68.9178) -> (-49.4403, 69.2684)
  line L23 (-49.4403, 69.2684) -> (-49.0588, 69.619)
  line L24 (-49.0588, 69.619) -> (-49.1187, 69.6961)
  arc A20 (-49.1187, 69.6961) -> (-49.2435, 69.8387) centre (-50.3783, 68.7188) ccw
  arc A21 (-49.2435, 69.8387) -> (-49.4908, 70.0838) centre (-60.4502, 58.7794) ccw
  arc A22 (-49.4908, 70.0838) -> (-49.7488, 70.3278) centre (-59.4752, 59.7852) ccw
  arc A23 (-49.7488, 70.3278) -> (-49.9351, 70.4876) centre (-52.0641, 67.8182) ccw
  arc A24 (-49.9351, 70.4876) -> (-50.698, 71.0097) centre (-53.8793, 65.5422) ccw
  arc A25 (-50.698, 71.0097) -> (-51.5212, 71.4089) centre (-53.7491, 65.766) ccw
  arc A26 (-51.5212, 71.4089) -> (-52.3959, 71.6801) centre (-53.7544, 65.7527) ccw
  arc A27 (-52.3959, 71.6801) -> (-53.3127, 71.8212) centre (-53.8245, 65.4466) ccw
  arc A28 (-53.3127, 71.8212) -> (-53.5357, 71.8337) centre (-53.6841, 67.195) ccw
  arc A29 (-53.5357, 71.8337) -> (-53.7872, 71.8375) centre (-53.7737, 64.3958) ccw
  arc A30 (-53.7872, 71.8375) -> (-54.0379, 71.8328) centre (-53.7737, 64.4287) ccw
  arc A31 (-54.0379, 71.8328) -> (-54.2587, 71.8195) centre (-53.8779, 67.3479) ccw
  arc A32 (-54.2587, 70.1206) -> (-54.8466, 70.011) centre (-53.685, 65.4098) ccw
  arc A33 (-54.8466, 70.011) -> (-55.4044, 69.8298) centre (-53.7721, 65.755) ccw
  arc A34 (-55.4044, 69.8298) -> (-55.9344, 69.5753) centre (-53.7639, 65.7344) ccw
  arc A35 (-55.9344, 69.5753) -> (-56.4394, 69.2471) centre (-53.5452, 65.3475) ccw
  arc A36 (-56.4394, 69.2471) -> (-56.6021, 69.1131) centre (-55.1906, 67.5645) ccw
  arc A37 (-56.6021, 69.1131) -> (-56.8494, 68.8817) centre (-47.9272, 59.5958) ccw
  arc A38 (-56.8494, 68.8817) -> (-57.0896, 68.6458) centre (-46.1793, 57.7765) ccw
  arc A39 (-57.0896, 68.6458) -> (-57.189, 68.5268) centre (-56.4605, 68.0191) ccw
  line L25 (-57.189, 68.5268) -> (-57.2288, 68.4697)
  line L26 (-57.2288, 68.4697) -> (-56.8503, 68.1124)
  line L27 (-56.8503, 68.1124) -> (-56.4719, 67.7551)
  line L28 (-56.4719, 67.7551) -> (-56.3945, 67.8485)
  arc A40 (-56.08, 68.1842) -> (-56.3945, 67.8485) centre (-53.4938, 65.4462) ccw
  arc A41 (-55.7342, 68.4703) -> (-56.08, 68.1842) centre (-53.7371, 65.7039) ccw
  arc A42 (-55.3591, 68.7046) -> (-55.7342, 68.4703) centre (-53.7966, 65.7862) ccw
  arc A43 (-54.9572, 68.886) -> (-55.3591, 68.7046) centre (-53.8154, 65.8213) ccw
  arc A44 (-53.9257, 69.0988) -> (-54.9572, 68.886) centre (-53.7527, 65.653) ccw
  arc A45 (-52.8891, 68.9868) -> (-53.9257, 69.0988) centre (-53.7593, 65.7856) ccw
  arc A46 (-51.9344, 68.5576) -> (-52.8891, 68.9868) centre (-53.7667, 65.7582) ccw
  arc A47 (-51.1412, 67.8487) -> (-51.9344, 68.5576) centre (-53.8865, 65.5753) ccw
  line L29 (-51.1412, 67.8487) -> (-51.064, 67.7555)
  line L30 (-51.064, 67.7555) -> (-50.6858, 68.113)
  line L31 (-50.6858, 68.113) -> (-50.3077, 68.4706)
  line L32 (-50.3077, 68.4706) -> (-50.3472, 68.5272)
  arc A48 (-50.3472, 68.5272) -> (-50.3748, 68.5616) centre (-50.6176, 68.3385) ccw
  arc A49 (-50.3748, 68.5616) -> (-50.4502, 68.6427) centre (-57.1721, 62.316) ccw
  arc A50 (-50.4502, 68.6427) -> (-50.5416, 68.7383) centre (-56.6313, 62.825) ccw
  arc A51 (-50.5416, 68.7383) -> (-50.6423, 68.8408) centre (-59.0523, 60.4741) ccw
  arc A52 (-50.6423, 68.8408) -> (-50.9283, 69.1069) centre (-54.2274, 65.2742) ccw
  arc A53 (-50.9283, 69.1069) -> (-51.2179, 69.3337) centre (-53.5264, 66.0886) ccw
  arc A54 (-51.2179, 69.3337) -> (-51.5267, 69.5325) centre (-53.5181, 66.1003) ccw
  arc A55 (-51.5267, 69.5325) -> (-51.8703, 69.7143) centre (-54.0251, 65.2263) ccw
  arc A56 (-51.8703, 69.7143) -> (-52.2117, 69.8601) centre (-53.6897, 65.9251) ccw
  arc A57 (-52.2117, 69.8601) -> (-52.5716, 69.9784) centre (-53.814, 65.594) ccw
  arc A58 (-52.5716, 69.9784) -> (-52.9406, 70.0666) centre (-53.8172, 65.5826) ccw
  arc A59 (-52.9406, 70.0666) -> (-53.3092, 70.1221) centre (-53.758, 65.8856) ccw
  arc A60 (-53.3092, 70.1221) -> (-53.5066, 70.1351) centre (-53.571, 67.6502) ccw
  arc A61 (-53.5066, 70.1351) -> (-53.7925, 70.1386) centre (-53.7766, 59.7306) ccw
  arc A62 (-53.7925, 70.1386) -> (-54.0758, 70.1343) centre (-53.7763, 59.5779) ccw
  arc A63 (-54.0758, 70.1343) -> (-54.2587, 70.1206) centre (-54.0197, 68.1585) ccw
  arc A64 (-53.9566, 68.4497) -> (-54.4448, 68.3648) centre (-53.6288, 65.1208) ccw
  arc A65 (-54.4448, 68.3648) -> (-54.8878, 68.2111) centre (-53.7904, 65.7631) ccw
  arc A66 (-54.8878, 68.2111) -> (-55.2884, 67.9865) centre (-53.8377, 65.8687) ccw
  arc A67 (-55.2884, 67.9865) -> (-55.6507, 67.6903) centre (-53.7254, 65.7048) ccw
  arc A68 (-55.6507, 67.6903) -> (-55.7671, 67.5728) centre (-52.8329, 64.7844) ccw
  arc A69 (-55.7671, 67.5728) -> (-55.878, 67.4511) centre (-52.882, 64.831) ccw
  arc A70 (-55.878, 67.4511) -> (-55.9747, 67.3383) centre (-50.1625, 62.4527) ccw
  arc A71 (-55.9747, 67.3383) -> (-55.9862, 67.3066) centre (-55.937, 67.3066) ccw
  arc A72 (-55.9862, 67.3066) -> (-55.9803, 67.293) centre (-55.9675, 67.3066) ccw
  arc A73 (-55.9803, 67.293) -> (-55.616, 66.95) centre (846.8811, 1025.8121) ccw
  arc A74 (-55.616, 66.95) -> (-55.2565, 66.6118) centre (406.487, 557.9133) ccw
  arc A75 (-55.2565, 66.6118) -> (-55.2311, 66.5959) centre (-55.2031, 66.6687) ccw
  arc A76 (-55.2311, 66.5959) -> (-55.2223, 66.5979) centre (-55.2282, 66.6034) ccw
  arc A77 (-55.2223, 66.5979) -> (-55.1959, 66.6269) centre (-55.9991, 67.3324) ccw
  arc A78 (-55.1959, 66.6269) -> (-55.1652, 66.664) centre (-55.7884, 67.1473) ccw
  arc A79 (-55.1652, 66.664) -> (-55.1316, 66.7092) centre (-56.3242, 67.5628) ccw
  arc A80 (-54.9296, 66.9414) -> (-55.1316, 66.7092) centre (-53.8047, 65.7595) ccw
  arc A81 (-54.6854, 67.1347) -> (-54.9296, 66.9414) centre (-53.7494, 65.7013) ccw
  arc A82 (-54.4086, 67.2816) -> (-54.6854, 67.1347) centre (-53.7382, 65.6842) ccw
  arc A83 (-54.1103, 67.376) -> (-54.4086, 67.2816) centre (-53.7414, 65.6918) ccw
  arc A84 (-53.9353, 67.3991) -> (-54.1103, 67.376) centre (-53.8862, 66.3529) ccw
  arc A85 (-53.7086, 67.4006) -> (-53.9353, 67.3991) centre (-53.8041, 64.6043) ccw
  arc A86 (-53.4824, 67.3837) -> (-53.7086, 67.4006) centre (-53.8042, 64.6022) ccw
  arc A87 (-53.3086, 67.3487) -> (-53.4824, 67.3837) centre (-53.6044, 66.3291) ccw
  arc A88 (-53.0433, 67.2446) -> (-53.3086, 67.3487) centre (-53.7437, 65.849) ccw
  arc A89 (-52.7884, 67.0901) -> (-53.0433, 67.2446) centre (-53.882, 65.5734) ccw
  arc A90 (-52.562, 66.8976) -> (-52.7884, 67.0901) centre (-53.8748, 65.5834) ccw
  arc A91 (-52.3821, 66.6806) -> (-52.562, 66.8976) centre (-53.6278, 65.8307) ccw
  arc A92 (-52.3821, 66.6806) -> (-52.3573, 66.6463) centre (-51.7286, 67.1265) ccw
  arc A93 (-52.3573, 66.6463) -> (-52.3339, 66.6182) centre (-52.0112, 66.9106) ccw
  arc A94 (-52.3339, 66.6182) -> (-52.3138, 66.5974) centre (-52.0055, 66.9158) ccw
  arc A95 (-52.3138, 66.5974) -> (-52.3051, 66.5957) centre (-52.3081, 66.6034) ccw
  arc A96 (-52.3051, 66.5957) -> (-52.2805, 66.611) centre (-52.3319, 66.6658) ccw
  arc A97 (-52.2805, 66.611) -> (-51.9201, 66.9494) centre (-549.7167, 596.8155) ccw
  arc A98 (-51.9201, 66.9494) -> (-51.555, 67.2925) centre (-1015.4894, 1092.5952) ccw
  arc A99 (-51.555, 67.2925) -> (-51.5493, 67.3057) centre (-51.5674, 67.3057) ccw
  arc A100 (-51.5493, 67.3057) -> (-51.5511, 67.3111) centre (-51.5584, 67.3057) ccw
  arc A101 (-51.5511, 67.3111) -> (-51.577, 67.3459) centre (-57.6783, 62.7919) ccw
  arc A102 (-51.577, 67.3459) -> (-51.6073, 67.3859) centre (-53.704, 65.7583) ccw
  arc A103 (-51.6073, 67.3859) -> (-51.6434, 67.4317) centre (-55.4356, 64.4141) ccw
  arc A104 (-51.6434, 67.4317) -> (-51.8307, 67.6391) centre (-53.3886, 66.043) ccw
  arc A105 (-51.8307, 67.6391) -> (-52.0622, 67.8451) centre (-54.1816, 65.2306) ccw
  arc A106 (-52.0622, 67.8451) -> (-52.3124, 68.0294) centre (-54.1914, 65.2185) ccw
  arc A107 (-52.3124, 68.0294) -> (-52.556, 68.1715) centre (-53.5902, 66.1179) ccw
  arc A108 (-52.556, 68.1715) -> (-52.7128, 68.2408) centre (-53.319, 66.6563) ccw
  arc A109 (-52.7128, 68.2408) -> (-52.9166, 68.3129) centre (-54.2275, 64.282) ccw
  arc A110 (-52.9166, 68.3129) -> (-53.1248, 68.3747) centre (-54.2334, 64.2639) ccw
  arc A111 (-53.1248, 68.3747) -> (-53.2958, 68.4121) centre (-53.5964, 66.626) ccw
  arc A112 (-53.2958, 68.4121) -> (-53.4493, 68.4322) centre (-53.6461, 66.331) ccw
  arc A113 (-53.4493, 68.4322) -> (-53.6452, 68.4469) centre (-53.9515, 63.0687) ccw
  arc A114 (-53.6452, 68.4469) -> (-53.8342, 68.4544) centre (-53.9543, 63.0201) ccw
  arc A115 (-53.8342, 68.4544) -> (-53.9566, 68.4497) centre (-53.8567, 67.4354) ccw
  arc A116 (-53.9849, 66.7348) -> (-54.24, 66.6166) centre (-53.7509, 65.8954) ccw
  arc A117 (-54.24, 66.6166) -> (-54.4464, 66.4226) centre (-53.7367, 65.8744) ccw
  arc A118 (-54.4464, 66.4226) -> (-54.5806, 66.1757) centre (-53.7487, 65.8837) ccw
  arc A119 (-54.5806, 66.1757) -> (-54.6266, 65.9041) centre (-53.8116, 65.9057) ccw
  arc A120 (-54.6266, 65.9041) -> (-54.5386, 65.5295) centre (-53.7788, 65.9058) ccw
  arc A121 (-54.5386, 65.5295) -> (-54.2936, 65.2285) centre (-53.7535, 65.9183) ccw
  arc A122 (-54.2936, 65.2285) -> (-53.9441, 65.0643) centre (-53.7598, 65.9102) ccw
  arc A123 (-53.9441, 65.0643) -> (-53.5637, 65.0719) centre (-53.77, 65.8637) ccw
  arc A124 (-53.5637, 65.0719) -> (-53.3439, 65.1598) centre (-53.8025, 65.9887) ccw
  arc A125 (-53.3439, 65.1598) -> (-53.1618, 65.2969) centre (-53.7393, 65.8743) ccw
  arc A126 (-53.1618, 65.2969) -> (-53.0247, 65.479) centre (-53.7393, 65.8743) ccw
  arc A127 (-53.0247, 65.479) -> (-52.9369, 65.6988) centre (-53.8536, 65.9376) ccw
  arc A128 (-52.9369, 65.6988) -> (-52.9297, 66.0834) centre (-53.733, 65.9062) ccw
  arc A129 (-52.9297, 66.0834) -> (-53.0974, 66.4344) centre (-53.7672, 65.8986) ccw
  arc A130 (-53.0974, 66.4344) -> (-53.4045, 66.6773) centre (-53.7775, 65.8904) ccw
  arc A131 (-53.4045, 66.6773) -> (-53.7859, 66.7602) centre (-53.7732, 65.8996) ccw
  arc A132 (-53.7859, 66.7602) -> (-53.8358, 66.7578) centre (-53.7746, 65.9967) ccw
  arc A133 (-53.8358, 66.7578) -> (-53.8914, 66.7521) centre (-53.7396, 65.5614) ccw
  arc A134 (-53.8914, 66.7521) -> (-53.9443, 66.7441) centre (-53.7479, 65.6266) ccw
  arc A135 (-53.9443, 66.7441) -> (-53.9849, 66.7348) centre (-53.8705, 66.3245) ccw
  arc A136 (-9.2413, 17.0805) -> (-8.2836, 17.2367) centre (-9.779, 23.3947) ccw
  arc A137 (-8.2836, 17.2367) -> (-7.3719, 17.5362) centre (-9.7146, 23.1295) ccw
  arc A138 (-7.3719, 17.5362) -> (-6.5197, 17.9755) centre (-9.7102, 23.1189) ccw
  arc A139 (-6.5197, 17.9755) -> (-5.739, 18.5475) centre (-9.8311, 23.3138) ccw
  arc A140 (-5.739, 18.5475) -> (-5.5697, 18.7002) centre (-8.7857, 22.0962) ccw
  arc A141 (-5.5697, 18.7002) -> (-5.3756, 18.8894) centre (-11.9553, 25.4432) ccw
  arc A142 (-5.3756, 18.8894) -> (-5.1963, 19.0746) centre (-11.7977, 25.2861) ccw
  arc A143 (-5.1963, 19.0746) -> (-5.0811, 19.2079) centre (-6.7042, 20.4934) ccw
  line L33 (-5.0811, 19.2079) -> (-5.0236, 19.2806)
  line L34 (-5.0236, 19.2806) -> (-5.4049, 19.6316)
  line L35 (-5.4049, 19.6316) -> (-5.7862, 19.9826)
  line L36 (-5.7862, 19.9826) -> (-5.8882, 19.8662)
  arc A144 (-6.4861, 19.284) -> (-5.8882, 19.8662) centre (-9.8321, 23.3187) ccw
  arc A145 (-7.1692, 18.8037) -> (-6.4861, 19.284) centre (-9.8382, 23.3261) ccw
  arc A146 (-7.9131, 18.4418) -> (-7.1692, 18.8037) centre (-9.7889, 23.2424) ccw
  arc A147 (-8.6921, 18.2113) -> (-7.9131, 18.4418) centre (-9.6579, 22.9072) ccw
  arc A148 (-9.2057, 18.1331) -> (-8.6921, 18.2113) centre (-9.7026, 23.1248) ccw
  arc A149 (-9.7322, 18.107) -> (-9.2057, 18.1331) centre (-9.7322, 23.4223) ccw
  arc A150 (-10.2587, 18.1331) -> (-9.7322, 18.107) centre (-9.7322, 23.4223) ccw
  arc A151 (-10.7723, 18.2113) -> (-10.2587, 18.1331) centre (-9.7618, 23.1248) ccw
  arc A152 (-11.5514, 18.4415) -> (-10.7723, 18.2113) centre (-9.8024, 22.9274) ccw
  arc A153 (-12.2933, 18.8021) -> (-11.5514, 18.4415) centre (-9.6926, 23.2091) ccw
  arc A154 (-12.9753, 19.2818) -> (-12.2933, 18.8021) centre (-9.6355, 23.3058) ccw
  arc A155 (-13.5761, 19.866) -> (-12.9753, 19.2818) centre (-9.5677, 23.3875) ccw
  line L37 (-13.5761, 19.866) -> (-13.6782, 19.9822)
  line L38 (-13.6782, 19.9822) -> (-14.0597, 19.6316)
  line L39 (-14.0597, 19.6316) -> (-14.4412, 19.281)
  line L40 (-14.4412, 19.281) -> (-14.3813, 19.2039)
  arc A156 (-14.3813, 19.2039) -> (-14.2565, 19.0613) centre (-13.1217, 20.1812) ccw
  arc A157 (-14.2565, 19.0613) -> (-14.0092, 18.8162) centre (-3.0498, 30.1206) ccw
  arc A158 (-14.0092, 18.8162) -> (-13.7512, 18.5722) centre (-4.0248, 29.1148) ccw
  arc A159 (-13.7512, 18.5722) -> (-13.5649, 18.4124) centre (-11.4359, 21.0818) ccw
  arc A160 (-13.5649, 18.4124) -> (-12.802, 17.8903) centre (-9.6207, 23.3578) ccw
  arc A161 (-12.802, 17.8903) -> (-11.9788, 17.4911) centre (-9.7509, 23.134) ccw
  arc A162 (-11.9788, 17.4911) -> (-11.1041, 17.2199) centre (-9.7456, 23.1473) ccw
  arc A163 (-11.1041, 17.2199) -> (-10.1873, 17.0788) centre (-9.6755, 23.4534) ccw
  arc A164 (-10.1873, 17.0788) -> (-9.9643, 17.0663) centre (-9.8159, 21.705) ccw
  arc A165 (-9.9643, 17.0663) -> (-9.7128, 17.0625) centre (-9.7263, 24.5042) ccw
  arc A166 (-9.7128, 17.0625) -> (-9.4621, 17.0672) centre (-9.7263, 24.4713) ccw
  arc A167 (-9.4621, 17.0672) -> (-9.2413, 17.0805) centre (-9.6221, 21.5521) ccw
  arc A168 (-9.2413, 18.7794) -> (-8.6534, 18.889) centre (-9.815, 23.4902) ccw
  arc A169 (-8.6534, 18.889) -> (-8.0956, 19.0702) centre (-9.7279, 23.145) ccw
  arc A170 (-8.0956, 19.0702) -> (-7.5656, 19.3247) centre (-9.7361, 23.1656) ccw
  arc A171 (-7.5656, 19.3247) -> (-7.0606, 19.6529) centre (-9.9548, 23.5525) ccw
  arc A172 (-7.0606, 19.6529) -> (-6.8979, 19.7869) centre (-8.3094, 21.3355) ccw
  arc A173 (-6.8979, 19.7869) -> (-6.6506, 20.0183) centre (-15.5728, 29.3042) ccw
  arc A174 (-6.6506, 20.0183) -> (-6.4104, 20.2542) centre (-17.3207, 31.1235) ccw
  arc A175 (-6.4104, 20.2542) -> (-6.311, 20.3732) centre (-7.0395, 20.8809) ccw
  line L41 (-6.311, 20.3732) -> (-6.2712, 20.4303)
  line L42 (-6.2712, 20.4303) -> (-6.6497, 20.7876)
  line L43 (-6.6497, 20.7876) -> (-7.0281, 21.1449)
  line L44 (-7.0281, 21.1449) -> (-7.1055, 21.0515)
  arc A176 (-7.42, 20.7158) -> (-7.1055, 21.0515) centre (-10.0062, 23.4538) ccw
  arc A177 (-7.7658, 20.4297) -> (-7.42, 20.7158) centre (-9.7629, 23.1961) ccw
  arc A178 (-8.1409, 20.1954) -> (-7.7658, 20.4297) centre (-9.7034, 23.1138) ccw